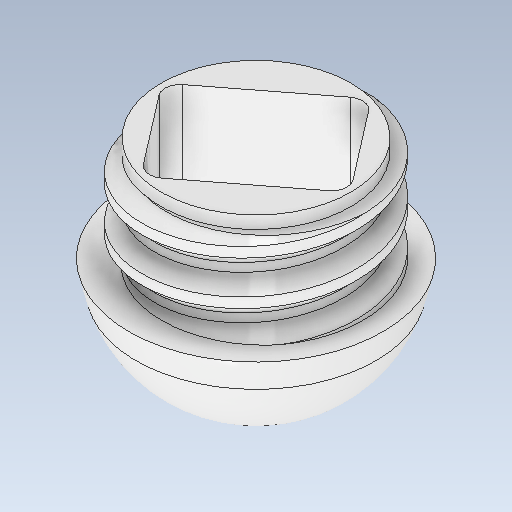
# Autodesk Inventor part: SmartEgg Shell
Saved by Autodesk Inventor 2020 (Build 240168000, 168)
## iProperties
Created: 2019-11-26
Part Number: SmartEgg Shell
Material: Generic
Document SubType Name: Modeling
Designer: Andrew
Density: 1 g/cm^3
Appearance: White
d0: 1.000 ul
d17: 1.000 ul
d18: 25.000 mm
d19: 50.000 mm
d20: 1.000 mm
d21: 17.000 mm
d22: 5.000 mm
d23: 2.000 mm
d24: 12.500 mm
d25: 0.250 mm
d26: 20.000 mm
d27: 3.000 mm
d28: 2.000 mm
d30: 1.000 mm
d32: 0.500 mm
d33: 0.500 mm
d35: 45.00 deg
d36: 0.250 mm
d37: 2.000 mm
d38: 2.000 mm
d41: 8.708 mm
d43: 3.000 ul
d44: 0.00 deg
d50: 8.708 mm
d52: 1.000 ul
d53: 0.00 deg
d61: 2.500 mm
d29: 68.767 mm
d39: 7.000 mm
Thread_Pitch: 4.354 mm
BATT_Width: 24.750 mm
PCB_Width: 22.850 mm
Author: Andrew
Autodesk Inventor part; units mm, degrees
ref_plane "YZ Plane" through (0, 0, 0) normal (1, 0, 0) x (0, 1, 0)
ref_plane "XZ Plane" through (0, 0, 0) normal (0, 1, 0) x (-1, 0, 0)
ref_plane "XY Plane" through (0, 0, 0) normal (0, 0, 1) x (1, 0, 0)
derived "SmartEgg Housing Main.ipt"
sketch "Sketch3" plane through (0, 0, 0) normal (0, 0, 1) x (1, 0, 0)
  line L0 (25.5, 9.75) -> (25.5, -9.25)
  line L1 (26.5, 11.5) -> (26.5, -11)
  line L2 (-26.5, -11) -> (-26.5, 11.5)
  line L3 (-8.0331, 6.4665) -> (-15.25, -6.0335)
  line L4 (-15.5, -5.9665) -> (-8.2831, 6.5335)
  line L5 (-26.5, 11.5) -> (-8.2831, 11.5)
  line L6 (-8.0331, 11.5) -> (26.5, 11.5)
  line L7 (-25.5, 9.75) -> (6.7169, 9.75)
  line L8 (6.9669, 9.75) -> (25.5, 9.75)
  line L9 (25.5, -9.25) -> (-0.25, -9.25)
  line L10 (-0.5, -9.25) -> (-25.5, -9.25)
  line L11 (26.5, -11) -> (-15.25, -11)
  line L12 (-15.5, -11) -> (-26.5, -11)
  line L13 (25.5, 0) -> (25.5, -1.75) construction
  line L14 (-25.5, -1.75) -> (-25.5, 0) construction
  line L15 (-25.5, -3.25) -> (-0.5, -3.25)
  line L16 (-0.5, -3.25) -> (-0.5, -4.25)
  line L17 (-0.5, -4.25) -> (-25.5, -4.25)
  line L18 (-25.5, -9.25) -> (-25.5, -4.25)
  line L19 (-25.5, -3.25) -> (-25.5, 9.75)
  line L20 (-8.1581, 11.5) -> (-8.1581, 6.5) construction
  line L21 (-8.1581, 6.5) -> (-15.375, -6) construction
  line L22 (-15.375, -6) -> (-15.375, -11) construction
  line L23 (-8.2831, 11.5) -> (-8.2831, 10.5)
  line L24 (-8.2831, 10.5) -> (6.7169, 10.5)
  line L25 (6.7169, 10.5) -> (6.7169, 9.75)
  line L26 (6.9669, 9.75) -> (6.9669, 10.75)
  line L27 (6.9669, 10.75) -> (-8.0331, 10.75)
  line L28 (-8.0331, 10.75) -> (-8.0331, 11.5)
  line L29 (-15.5, -11) -> (-15.5, -10)
  line L30 (-15.5, -10) -> (-0.5, -10)
  line L31 (-0.5, -10) -> (-0.5, -9.25)
  line L32 (-0.25, -9.25) -> (-0.25, -10.25)
  line L33 (-0.25, -10.25) -> (-15.25, -10.25)
  line L34 (-15.25, -10.25) -> (-15.25, -11)
  line L35 (-8.2831, 10.5) -> (-8.2831, 6.5335)
  line L36 (-8.0331, 6.4665) -> (-8.0331, 10.75)
  line L37 (-15.5, -10) -> (-15.5, -5.9665)
  line L38 (-15.25, -6.0335) -> (-15.25, -10.25)
  line L39 (6.7169, 9.75) -> (6.7169, 6.5335)
  line L40 (6.7169, 6.5335) -> (-0.5, -5.9665)
  line L41 (-0.5, -5.9665) -> (-0.5, -9.25)
  line L42 (-0.25, -9.25) -> (-0.25, -6.0335)
  line L43 (-0.25, -6.0335) -> (6.9669, 6.4665)
  line L44 (6.9669, 6.4665) -> (6.9669, 9.75)
  line L45 (-0.375, -11) -> (-0.375, -6) construction
  line L46 (-0.375, -6) -> (6.8419, 6.5) construction
  line L47 (6.8419, 6.5) -> (6.8419, 11.5) construction
  line L48 (11.5, -9.25) -> (16.5, -9.25)
  line L49 (16.5, -9.25) -> (14, -6.75)
  line L50 (14, -6.75) -> (11.5, -6.75)
  line L51 (11.5, -6.75) -> (11.5, -9.25)
  point P0 (0, 0)
derived "SmartEgg Housing Cap.ipt"
sketch "Housing Largest Area" plane through (0, -9.787, -13.5347) normal (0, 0.8032373, -0.5956591) x (0, 0.5956591, 0.8032373)
  line L0 (29.2004, 26.5) -> (28.5488, 26.5)
  line L1 (16.8502, 26.5) -> (16.8502, -26.5)
  line L2 (16.8502, -26.5) -> (33.7004, -26.5)
  line L3 (33.7004, -26.5) -> (33.7004, 22)
  line L4 (10.149, -26.5) -> (23.5514, -26.5) construction
  line L5 (23.5514, 26.5) -> (10.149, 26.5) construction
  line L6 (10.9744, 20.5) -> (9.2955, 20.5) construction
  line L7 (9.2955, 20.5) -> (9.2955, 24.5) construction
  ellipse E0 centre (7.6167, 24.5) end of major axis (9.2955, 24.5) minor radius 1 (9.2955, 24.5) -> (7.6167, 25.5) ccw construction
  line L8 (7.6167, 25.5) -> (1.6516, 25.5) construction
  line L9 (1.6516, 25.5) -> (1.6516, -0.25) construction
  line L10 (1.6516, -0.25) -> (0.6509, -0.25) construction
  line L11 (0.6509, -0.25) -> (0.6509, -15.25) construction
  line L12 (0.6509, -15.25) -> (0, -15.25) construction
  line L13 (0, -15.25) -> (0, 24.5) construction
  arc A0 (2, 26.5) -> (0, 24.5) centre (2, 24.5) ccw construction
  line L14 (2, 26.5) -> (16.4305, 26.5) construction
  line L15 (16.4305, 26.5) -> (16.4305, 25.5) construction
  line L16 (16.4305, 25.5) -> (13.4926, 25.5) construction
  line L17 (13.4926, 25.5) -> (13.4926, 22.4142) construction
  ellipse E1 centre (11.8138, 22.4142) end of major axis (13.4926, 22.4142) minor radius 1 (13.0009, 21.7071) -> (13.4926, 22.4142) ccw construction
  line L18 (13.0009, 21.7071) -> (10.9744, 20.5) construction
  arc A1 (33.7004, 24.5) -> (31.7004, 26.5) centre (31.7004, 24.5) ccw construction
  line L19 (33.7004, 24.5) -> (33.7004, -8.0331) construction
  line L20 (33.7004, -8.0331) -> (33.0495, -8.0331) construction
  line L21 (33.0495, -8.0331) -> (33.0495, 6.9669) construction
  line L22 (33.0495, 6.9669) -> (32.0488, 6.9669) construction
  line L23 (32.0488, 6.9669) -> (32.0488, 25.5) construction
  line L24 (32.0488, 25.5) -> (20.6275, 25.5) construction
  line L25 (20.6275, 25.5) -> (20.6275, 26.5) construction
  line L26 (20.6275, 26.5) -> (31.7004, 26.5) construction
  arc A2 (33.7004, 22) -> (29.2004, 26.5) centre (29.2004, 22) ccw
  arc A3 (32.0488, 22) -> (28.5488, 25.5) centre (28.5488, 22) ccw
  line L27 (32.0488, 22) -> (33.7004, 22)
  line L28 (28.5488, 25.5) -> (28.5488, 26.5)
  line L29 (28.5488, 26.5) -> (16.8502, 26.5)
  point P0 (16.7013, 0)
  point P1 (16.8502, 0)
sketch "ESP32 Feather" plane through (0, 0, 0) normal (0, 0, 1) x (1, 0, 0)
  line L0 (-25.5, 0) -> (25.5, 0)
  line L1 (25.5, 0) -> (25.5, -1.75)
  line L2 (25.5, -1.75) -> (-25.5, -1.75)
  line L3 (-25.5, -1.75) -> (-25.5, 0)
  line L4 (0, 0) -> (-25.5, 0)
  line L5 (-25.5, 0) -> (-25.5, 0.8)
  line L6 (-25.5, 0.8) -> (0, 0.8)
  line L7 (0, 0.8) -> (0, 0)
  line L8 (-0.9, 0.8) -> (-18.55, 0.8)
  line L9 (-18.55, 0.8) -> (-18.55, 3.15)
  line L10 (-18.55, 3.15) -> (-0.9, 3.15)
  line L11 (-0.9, 3.15) -> (-0.9, 0.8)
  line L12 (10.75, 0) -> (18.75, 0)
  line L13 (18.75, 0) -> (18.75, 5.5)
  line L14 (18.75, 5.5) -> (10.75, 5.5)
  line L15 (10.75, 5.5) -> (10.75, 0)
  line L16 (25.6, 0) -> (19.95, 0)
  line L17 (19.95, 0) -> (19.95, 2.5)
  line L18 (19.95, 2.5) -> (25.6, 2.5)
  line L19 (25.6, 2.5) -> (25.6, 0)
  point P0 (0, 0)
  point P1 (0, 0)
  point P2 (19.95, 0)
sketch "Shell Sketch" plane through (0, -9.787, -13.5347) normal (0, 0.8032373, -0.5956591) x (0, 0.5956591, 0.8032373)
  arc A0 (40.7438, -16.765) -> (29.159, 32.4326) centre (-7.0434, -2.0549) ccw
  arc A1 (16.8502, -34.4099) -> (29.3502, -31.0606) centre (16.8502, -9.4099) ccw construction
  line L0 (16.8502, -34.4099) -> (16.8502, -31.0606) construction
  line L1 (16.8502, 9.75) -> (35.7004, 9.75)
  line L2 (16.8502, 26.5) -> (16.8502, -26.5) construction
  line L3 (33.7004, -26.5) -> (34.4025, -27.2121) construction
  arc A2 (29.159, 32.4326) -> (16.8502, 37.7068) centre (16.8502, 20.7068) ccw
  line L4 (16.8502, 37.7068) -> (16.8502, 34.849)
  line L5 (16.8502, 34.849) -> (21.8502, 34.849)
  arc A3 (27.7109, 31.0531) -> (21.8502, 34.849) centre (16.8502, 20.7068) ccw
  arc A4 (37.5734, 15.6465) -> (27.7109, 31.0531) centre (-7.0434, -2.0549) ccw
  arc A5 (33.7004, 22) -> (29.2004, 26.5) centre (29.2004, 22) ccw construction
  line L6 (35.7004, 9.75) -> (35.7004, -11.0606)
  line L7 (35.7004, -11.0606) -> (42.1389, -11.0606)
  line L8 (38.7004, 9.75) -> (38.7004, -10.8106)
  line L9 (38.7004, -10.8106) -> (42.184, -10.8106)
  line L10 (16.8502, -31.0606) -> (29.3502, -31.0606)
  arc A6 (29.3502, -31.0606) -> (40.7438, -16.765) centre (16.8502, -9.4099) ccw
  line L11 (16.8502, -31.0606) -> (16.8502, 9.75)
  line L12 (33.7004, -26.5) -> (33.7004, 22) construction
  line L13 (19.9774, 10.75) -> (16.7013, 10.75) construction
  arc A7 (38.7004, 9.75) -> (37.5734, 15.6465) centre (22.7111, 9.75) ccw
  point P0 (16.7013, 0)
  point P1 (38.7004, 12.4883)
  dimension "d18" = 25
  dimension "d19" = 50
  dimension "d20" = 1
  dimension "d21" = 17
  dimension "d22" = 5
  dimension "d23" = 2
  dimension "d24" = 12.5
  dimension "d25" = 0.25
  dimension "d26" = 20
  dimension "d27" = 3
  dimension "d28" = 2
  dimension "d29" = 68.7674
  dimension "d30" = 1
  constraints: 22 end point, 19 point on circle, 7 centre point, 7 line through centre, 6 perpendicular, 6 tangent, 4 collinear, 4 vertical, 2 concentric, 2 point on line, 1 coincident, 1 horizontal
  measures "d18" radius of A1
  measures "d19" radius of A0
  measures "d20" distance of L3.start L3.end
  measures "d21" radius of A2
  measures "d22" distance of L4.end L5.end
  measures "d23" radial gap between concentric circles of A0 A4
  measures "d24" distance of L0.end L10.end
  measures "d25" distance between parallel lines of L7 L9
  measures "d26" distance between parallel lines of L10 L7
  measures "d27" distance between parallel lines of L8 L6
  measures "d28" distance between parallel lines of L12 L6
  measures "d29" distance from line of L10 L4.start
  measures "d30" distance between parallel lines of L1 L13
sketch "Thread Sketch" plane through (0, -9.787, -13.5347) normal (0, 0.8032373, -0.5956591) x (0, 0.5956591, 0.8032373)
  line L0 (35.7004, 9.75) -> (35.7004, -11.0606) construction
  line L1 (38.7004, 9.75) -> (38.7004, -10.8106) construction
  line L2 (35.7004, 9.75) -> (38.2004, 7.25)
  line L3 (38.2004, 7.25) -> (38.2004, 5.25)
  line L4 (38.2004, 5.25) -> (35.7004, 2.75)
  line L5 (35.7004, 2.75) -> (35.7004, 9.75)
  line L6 (38.7004, 5.3964) -> (36.2004, 2.8964)
  line L7 (36.2004, 2.8964) -> (36.2004, 0.8964)
  line L8 (36.2004, 0.8964) -> (38.7004, -1.6036)
  line L9 (38.7004, -1.6036) -> (38.7004, 5.3964)
  line L10 (38.2004, 6.25) -> (35.7004, 6.25) construction
  line L11 (36.2004, 1.8964) -> (38.7004, 1.8964) construction
  point P0 (16.7013, 0)
  dimension "d32" = 0.5
  dimension "d33" = 0.5
  dimension "d35" = 45
  dimension "d36" = 0.25
  dimension "d37" = 2
  dimension "d38" = 2
  dimension "d39" = 7
  dimension "Thread_Pitch" = 4.354
  constraints: 20 end point, 4 midpoint, 3 parallel, 2 horizontal, 2 point on line, 2 other
  measures "d32" distance between parallel lines of L1 L3
  measures "d33" distance between parallel lines of L0 L7
  measures "d35" angle of L0 L4
  measures "d36" distance between parallel lines of L6 L4
  measures "d37" distance of L2.end L3.end
  measures "d38" distance of L6.end L7.end
  measures "d39" distance of L4.end L0.start
revolve "Revolution1" add sketch "Shell Sketch" angle 360 about axis through (-31.0606, 0.25, 0) along (1, 0, 0) contours A6 L10 L11 L1 L6 L7 A0
coil "Coil1" sketch "Thread Sketch" operation add axis through (-31.0606, 0.25, 0) along (-1, 0, 0) pitch 8.708 turns 3 hand right separate body contours L2 L3 L4 L5
coil "Coil2" sketch "Thread Sketch" operation add axis through (-31.0606, 0.25, 0) along (1, 0, 0) pitch 8.708 turns 1 hand right bodies 2 contours L2 L3 L4 L5
sketch "Thread Mask" plane through (0, -9.787, -13.5347) normal (0, 0.8032373, -0.5956591) x (0, 0.5956591, 0.8032373)
  line L0 (38.7004, 7.25) -> (35.7004, 7.25)
  line L1 (35.7004, 7.25) -> (35.7004, -11.0606)
  line L2 (35.7004, -11.0606) -> (38.7004, -11.0606)
  line L3 (38.7004, -11.0606) -> (38.7004, 7.25)
  line L4 (35.7004, 9.75) -> (35.7004, -11.0606) construction
  line L5 (38.7004, 9.75) -> (38.7004, -10.8106) construction
  point P0 (16.7013, 0)
  dimension "d61" = 2.5
  constraints: 8 end point, 2 parallel, 1 collinear, 1 horizontal, 1 perpendicular
  measures "d61" distance from line of L4.start L0
revolve "Revolution4" cut sketch "Thread Mask" angle 360 about axis through (-31.0606, 0.25, 0) along (1, 0, 0) keep common part bodies 2
combine bodies "Combine1" operation type add bodies to combine 1 2
sketch "Sketch10" plane through (9.75, 0.25, 0) normal (1, 0, 0) x (0, 0, -1)
  line L0 (-11.875, -11.5) -> (11.875, -11.5)
  line L1 (14.875, -8.5) -> (14.875, 8.5)
  line L2 (11.875, 11.5) -> (-11.875, 11.5)
  line L3 (-14.875, 8.5) -> (-14.875, -8.5)
  line L4 (-14.875, 0) -> (14.875, 0) construction
  arc A0 (-11.875, 11.5) -> (-14.875, 8.5) centre (-11.875, 8.5) ccw
  arc A1 (14.875, 8.5) -> (11.875, 11.5) centre (11.875, 8.5) ccw
  arc A2 (11.875, -11.5) -> (14.875, -8.5) centre (11.875, -8.5) ccw
  arc A3 (-14.875, -8.5) -> (-11.875, -11.5) centre (-11.875, -8.5) ccw
  point P0 (0, -0.25)
  point P1 (14.875, 11.5)
  point P2 (-14.875, 11.5)
  point P3 (0, -11.25)
  point P4 (0, -11.25)
  point P5 (0, -11.25)
  point P6 (0, 11.25)
  point P7 (0, 11.25)
  point P8 (0, 11.25)
  point P9 (0, 0)
  point P10 (0, 0)
  point P11 (0, 0)
  point P12 (0, 0)
  dimension "d64" = 0.25
  dimension "d65" = 29.75
  dimension "d66" = 3
  constraints: 10 end point, 8 point on circle, 8 tangent, 4 centre point, 4 point on line, 3 equal radius, 3 midpoint, 2 parallel, 1 coincident, 1 horizontal, 1 perpendicular
  measures "d64" distance from line of L0 point (0, -11.25)
  measures "d65" distance of point (14.875, 11.5) point (-14.875, 11.5)
  measures "d66" radius of A0
sketch "Sketch11" plane through (0, 0, 0) normal (0, 0, 1) x (1, 0, 0)
  line L0 (9.75, 19.1002) -> (9.75, -18.6002) projected
  line L1 (9.75, 0.25) -> (-26.5, 0.25)
  line L2 (-26.5, -11) -> (-26.5, 11.5) construction
  point P0 (0, 0)
  dimension "d67" = 36.25
  constraints: 2 end point, 2 midpoint, 1 horizontal
  measures "d67" distance of L1.start L1.end
extrude "Extrusion1" cut sketch "Sketch10" against normal blind 36.25 bodies 1
fillet "Fillet1" radius 2.25 8 edges at (-26.5, 10.8713, 13.9963) (-26.5, 11.75, 0) (-26.5, 10.8713, -13.9963) (-26.5, 0.25, -14.875) (-26.5, -10.3713, -13.9963) (-26.5, -11.25, 0) (-26.5, -10.3713, 13.9963) (-26.5, 0.25, 14.875)
sketch "Vent Lookup" plane through (0, -9.787, -13.5347) normal (0, 0.8032373, -0.5956591) x (0, 0.5956591, 0.8032373)
  arc A0 (40.7438, -16.765) -> (29.159, 32.4326) centre (-7.0434, -2.0549) ccw projected
  line L0 (39.0795, 17.25) -> (16.8502, 7.9458)
  line L1 (16.8502, 26.5) -> (16.8502, -26.5) construction
  line L2 (19.9774, 10.75) -> (16.7013, 10.75) construction
  point P0 (16.7013, 0)
  dimension "d71" = 6.5
  constraints: 2 end point, 1 line through centre, 1 point on circle, 1 point on line
  measures "d71" distance from line of L2 L0.start
ref_plane "Vent Plane" through (17.25, 13.4911, 17.8554) normal (-0.3860978, -0.5494704, -0.7409526) x (0.8182033, -0.574929, 0)
ref_plane "Work Plane2" through (0, -9.787, -13.5347) normal (0, 0.8032373, -0.5956591) x (0, 0.5956591, 0.8032373)
equation "\"d38\" = d37"
equation "\"d41\" = 2 * Thread_Pitch"
equation "\"d50\" = 2 * Thread_Pitch"
equation "\"d68\" = d67"
body "Solid1"
body "Solid3"
